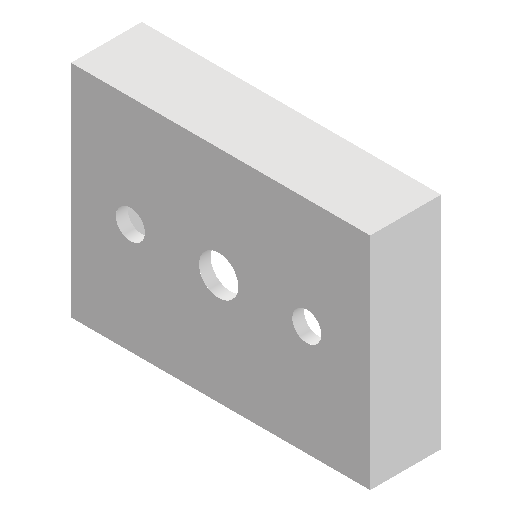
# Autodesk Inventor part: estructura_sensor_chumacera
Saved by Autodesk Inventor 2025 (Build 290162000, 162)
## iProperties
Created: 2026-02-02
Part Number: estructura_sensor_chumacera
Material: Genérico
Document SubType Name: Modeling
Designer: HP
Density: 1 g/cm^3
Appearance: Valor por defecto
Author: HP
Autodesk Inventor part; units mm, degrees
ref_plane "YZ Plane" through (0, 0, 0) normal (1, 0, 0) x (0, 1, 0)
ref_plane "XZ Plane" through (0, 0, 0) normal (0, 1, 0) x (-1, 0, 0)
ref_plane "XY Plane" through (0, 0, 0) normal (0, 0, 1) x (1, 0, 0)
sketch "Boceto1" plane through (0, 0, 0) normal (0, 0, 1) x (1, 0, 0)
  arc A0 (-1.75, 0) -> (-0.6468, -1.6261) centre (0, 0) ccw projected
  line L0 (-1.75, 0) -> (-1.75, 5.2862) projected
  arc A1 (-0.6468, 6.9123) -> (-1.75, 5.2862) centre (0, 5.2862) ccw projected
  line L1 (-0.6468, 6.9123) -> (12.6254, 12.1912) projected
  arc A2 (12.6254, 12.1912) -> (13.6116, 12.956) centre (11.7938, 14.2819) ccw projected
  arc A3 (41.8884, 12.956) -> (13.6116, 12.956) centre (27.75, 2.6431) ccw projected
  arc A4 (41.8884, 12.956) -> (42.8746, 12.1912) centre (43.7062, 14.2819) ccw projected
  line L2 (42.8746, 12.1912) -> (56.1468, 6.9123) projected
  arc A5 (57.25, 5.2862) -> (56.1468, 6.9123) centre (55.5, 5.2862) ccw projected
  line L3 (57.25, 5.2862) -> (57.25, 0) projected
  arc A6 (56.1468, -1.6261) -> (57.25, 0) centre (55.5, 0) ccw projected
  line L4 (56.1468, -1.6261) -> (42.8746, -6.905) projected
  arc A7 (42.8746, -6.905) -> (41.8884, -7.6698) centre (43.7062, -8.9957) ccw projected
  arc A8 (13.6116, -7.6698) -> (41.8884, -7.6698) centre (27.75, 2.6431) ccw projected
  arc A9 (13.6116, -7.6698) -> (12.6254, -6.905) centre (11.7938, -8.9957) ccw projected
  line L5 (12.6254, -6.905) -> (-0.6468, -1.6261) projected
  circle A10 centre (50.15, 2.6431) radius 3.7 projected
  circle A11 centre (5.35, 2.6431) radius 3.7 projected
  arc A12 (44.3063, 7.4106) -> (11.1937, 7.4106) centre (27.75, 2.6431) ccw projected
  arc A13 (11.1937, 7.4106) -> (11.3578, 5.7658) centre (13.3357, 6.7938) ccw projected
  arc A14 (11.3578, -0.4796) -> (11.3578, 5.7658) centre (5.35, 2.6431) ccw projected
  arc A15 (11.3578, -0.4796) -> (11.1937, -2.1244) centre (13.3357, -1.5076) ccw projected
  arc A16 (11.1937, -2.1244) -> (44.3063, -2.1244) centre (27.75, 2.6431) ccw projected
  arc A17 (44.3063, -2.1244) -> (44.1422, -0.4796) centre (42.1643, -1.5076) ccw projected
  arc A18 (44.1422, 5.7658) -> (44.1422, -0.4796) centre (50.15, 2.6431) ccw projected
  arc A19 (44.1422, 5.7658) -> (44.3063, 7.4106) centre (42.1643, 6.7938) ccw projected
  line L6 (-6.75, 27.6431) -> (63.25, 27.6431)
  line L7 (63.25, 27.6431) -> (63.25, -22.3569)
  line L8 (63.25, -22.3569) -> (-6.75, -22.3569)
  line L9 (-6.75, -22.3569) -> (-6.75, 27.6431)
  line L10 (-6.75, 2.6431) -> (63.25, 2.6431) construction
  point P0 (-1.75, 2.6431)
  dimension "d0" = 70
  dimension "d1" = 50
  dimension "d2" = 5
  dimension "d3" = 6
  constraints: 10 end point, 3 midpoint, 2 parallel, 1 horizontal, 1 perpendicular, 1 point on line
  measures "d0" distance of L7.end L8.end
  measures "d1" distance of L6.end L7.end
  measures "d2" distance from line of L9 point (-1.75, 2.643)
  measures "d3" distance between parallel lines of L3 L7
extrude "Extrusión1" add sketch "Boceto1" along normal blind 3 contours L0 A1 L1 A2 A3 A4 L2 A5 L3 A6 L4 A7 A8 A9 L5 A0 | A19 A18 A17 A16 A15 A14 A13 A12 | L6 L7 L8 L9
sketch "Boceto2" plane through (0, 0, 0) normal (0, 0, -1) x (-1, 0, 0)
  circle A0 centre (-27.75, 2.6431) radius 5 projected
  line L0 (6.75, -22.3569) -> (-63.25, -22.3569) projected
  line L1 (6.75, 27.6431) -> (6.75, -22.3569) projected
  line L2 (-63.25, 27.6431) -> (6.75, 27.6431) projected
  line L3 (-63.25, -22.3569) -> (-63.25, 27.6431) projected
  circle A1 centre (-5.35, 2.6431) radius 3.7 projected
  circle A2 centre (-50.15, 2.6431) radius 3.7 projected
  line L4 (-66.25, -25.3569) -> (9.75, -25.3569)
  line L5 (9.75, -25.3569) -> (9.75, 30.6431)
  line L6 (9.75, 30.6431) -> (-66.25, 30.6431)
  line L7 (-66.25, 30.6431) -> (-66.25, -25.3569)
  point P0 (0, 0)
  dimension "d6" = 3
  constraints: 8 end point, 3 other
  measures "d6" distance between parallel lines of L0 L4
extrude "Extrusión2" cut sketch "Boceto2" against normal through all contours A0
sketch "Boceto4" plane through (0, 0, 0) normal (0, 0, -1) x (-1, 0, 0)
  circle A0 centre (-27.75, 2.6431) radius 5 projected
  line L0 (6.75, -22.3569) -> (-63.25, -22.3569) projected
  line L1 (6.75, 27.6431) -> (6.75, -22.3569) projected
  line L2 (-63.25, 27.6431) -> (6.75, 27.6431) projected
  line L3 (-63.25, -22.3569) -> (-63.25, 27.6431) projected
  circle A1 centre (-5.35, 2.6431) radius 3.7 projected
  circle A2 centre (-50.15, 2.6431) radius 3.7 projected
  line L4 (9.75, -25.3569) -> (-66.25, -25.3569)
  line L5 (-66.25, -25.3569) -> (-66.25, 30.6431)
  line L6 (-66.25, 30.6431) -> (9.75, 30.6431)
  line L7 (9.75, 30.6431) -> (9.75, -25.3569)
  point P0 (0, 0)
  dimension "d9" = 3
  constraints: 8 end point, 3 other
  measures "d9" distance between parallel lines of L1 L7
extrude "Extrusión3" add sketch "Boceto4" along normal blind 15 and the other way blind 3 contours L4 L5 L6 L7
